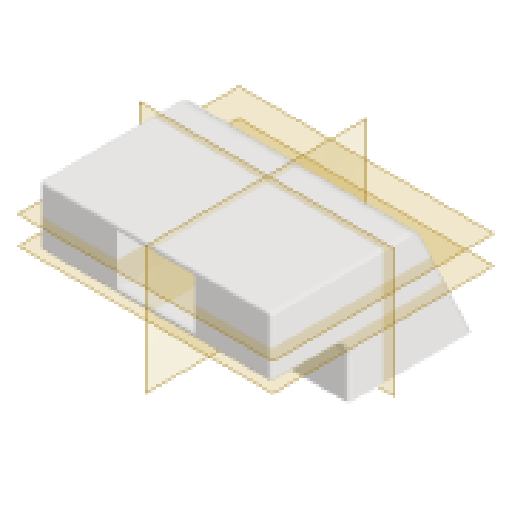
# Autodesk Inventor part: Вторая часть петли
Saved by Autodesk Inventor 2023.2 (Build 272271030, 271C)
## iProperties
Created: 2025-05-06
Part Number: Вторая часть петли
Material: Типовые
Document SubType Name: Modeling
Designer: Олег Коноваленко
Density: 1 g/cm^3
Appearance: По умолчанию
Author: Олег Коноваленко
Autodesk Inventor part; units mm, degrees
sketch "Эскиз1" plane through (0, 0, 0) normal (1, 0, 0) x (0, 1, 0)
  line L0 (-37.5, -57.5) -> (-37.5, 22.5)
  line L1 (-37.5, -57.5) -> (37.5, -22.5)
  line L2 (37.5, -22.5) -> (37.5, 22.5)
  line L3 (37.5, 22.5) -> (-37.5, 22.5)
  line L4 (37.5, -22.5) -> (-37.5, -22.5)
  line L5 (37.5, 22.5) -> (-37.5, -22.5) construction
  line L6 (37.5, -22.5) -> (-37.5, 22.5) construction
  line L7 (-52.5, 0) -> (52.5, 0) projected
  line L8 (0, 168.3234) -> (0, -95.1372) construction
  line L9 (18, 130.6862) -> (18, 46.6862) construction
  line L10 (37.5, 72.5) -> (37.5, 22.5)
  line L11 (-1.5, 72.5) -> (-1.5, 22.5)
  circle A0 centre (27.5, -16.1314) radius 10
  circle A1 centre (-11.5, 32.5) radius 10
  line L12 (37.5, 72.5) -> (-1.5, 72.5)
  point P0 (0, 0)
  point P1 (0, 0)
  point P2 (0, 0)
  point P3 (18, 88.6862)
  point P4 (0, 22.5)
  point P5 (19.7902, -22.5)
  point P6 (35.2098, -22.5)
  point P7 (37.5, -16.1314)
  point P8 (31.7289, -25.1932)
  point P9 (-1.5, 32.5)
  point P10 (-11.5, 22.5)
  dimension "d2" = 75
  dimension "d3" = 45
  dimension "d4" = 80
  dimension "d10" = 20
  dimension "d13" = 20
  dimension "d16" = 39
  dimension "d17" = 50
  constraints: 22 end point, 5 perpendicular, 4 midpoint, 4 tangent, 3 point on line, 3 vertical, 2 centre point, 2 other
  measures "d2" distance of L2.end L0.end
  measures "d3" distance of L1.end L2.end
  measures "d4" distance of L0.start L0.end
  measures "d10" diameter of A0
  measures "d13" diameter of A1
  measures "d16" distance of L11.start L10.start
  measures "d17" distance between parallel lines of L3 L12
extrude "Выдавливание2" add sketch "Эскиз1" along normal mid plane 150 contours L0 L4 A0 L1 | L0 L7 L2 A0 L4 | A0 L4 | L0 L3 L2 L7 | A0 L4 | A1 L11 L3 | L3 L11 L12 L10
fillet "Сопряжение1" radius 2 12 edges at (75, -1.5, 52.5) (75, -4.4289, 25.4289) (75, -24.5, 22.5) (75, 35.9347, -21.5031) (75, -2.8856, -41.3466) (75, 37.5, 28.1843) (-75, 35.9347, -21.5031) (-75, 37.5, 28.1843) (-75, -1.5, 52.5) (-75, -4.4289, 25.4289) (-75, -24.5, 22.5) (-75, -2.8856, -41.3466)
ref_plane "РабПлоскость1" through (-73, 18, 72.5) normal (0, 1, 0) x (1, 0, 0)
sketch "Эскиз7" plane through (-73, -1.5, 72.5) normal (0, 0, 1) x (1, 0, 0)
  line L0 (49, 34.5) -> (49, 4.5) construction
  line L1 (97, 4.5) -> (49, 4.5) construction
  line L2 (97, 34.5) -> (97, 4.5) construction
  line L3 (49, 34.5) -> (97, 34.5) construction
  line L4 (48.5, 4) -> (97.5, 4)
  line L5 (97.5, 4) -> (97.5, 35)
  line L6 (97.5, 35) -> (48.5, 35)
  line L7 (48.5, 35) -> (48.5, 4)
  line L8 (48.5, 4) -> (97.5, 35) construction
  line L9 (97.5, 4) -> (48.5, 35) construction
  point P0 (73, 1.5)
  point P1 (73, 19.5)
  dimension "d24" = 0.5
  dimension "d25" = 0.5
  dimension "d26" = 0.5
  dimension "d27" = 0.5
  constraints: 12 end point, 2 midpoint, 2 parallel, 1 horizontal, 1 perpendicular
  measures "d24" distance between parallel lines of L2 L5
  measures "d25" distance between parallel lines of L3 L6
  measures "d26" distance between parallel lines of L4 L1
  measures "d27" distance between parallel lines of L7 L0
extrude "Выдавливание6" cut sketch "Эскиз7" against normal blind 42.5
ref_plane "РабПлоскость2" through (24, 3, 30) normal (1, 0, 0) x (0, 1, 0)
ref_plane "РабПлоскость3" through (24, 3, 35.5) normal (1, 0, 0) x (0, 1, 0)
ref_plane "РабПлоскость4" through (-24, 3, 35.5) normal (-1, 0, 0) x (0, 0, 1)
fillet "Сопряжение2" radius 2 8 edges at (74.4142, 36.9142, 72.5) (75, 18, 72.5) (74.4142, -0.9142, 72.5) (0, -1.5, 72.5) (-74.4142, -0.9142, 72.5) (-75, 18, 72.5) (-74.4142, 36.9142, 72.5) (0, 37.5, 72.5)
chamfer "Фаска1" distance 1 angle 45 4 edges at (0, 33.5, 72.5) (-24.5, 18, 72.5) (0, 2.5, 72.5) (24.5, 18, 72.5)
sketch "Эскиз14" plane through (-73, -37.5, -57.5) normal (0, -1, 0) x (1, 0, 0)
  circle A0 centre (133, 70) radius 1.15
  line L0 (148, 78) -> (148, 2.2071) projected
  line L1 (0, 80) -> (146, 80) projected
  circle A1 centre (133, 55) radius 1.15
  circle A2 centre (133, 40) radius 1.15
  circle A3 centre (133, 25) radius 1.15
  circle A4 centre (133, 10) radius 1.15
  circle A5 centre (93, 70) radius 1.15
  circle A6 centre (93, 55) radius 1.15
  circle A7 centre (93, 40) radius 1.15
  circle A8 centre (93, 25) radius 1.15
  circle A9 centre (93, 10) radius 1.15
  circle A10 centre (53, 70) radius 1.15
  circle A11 centre (53, 55) radius 1.15
  circle A12 centre (53, 40) radius 1.15
  circle A13 centre (53, 25) radius 1.15
  circle A14 centre (53, 10) radius 1.15
  circle A15 centre (13, 70) radius 1.15
  circle A16 centre (13, 55) radius 1.15
  circle A17 centre (13, 40) radius 1.15
  circle A18 centre (13, 25) radius 1.15
  circle A19 centre (13, 10) radius 1.15
  point P0 (73, 57.5)
  dimension "d62" = 2.3
  dimension "d63" = 15
  dimension "d64" = 10
  dimension "d67" = 15
  dimension "d74" = 40
  constraints: 20 centre point, 1 horizontal, 1 vertical, 38 other
  measures "d62" diameter of A0
  measures "d63" distance from line of L0 A0.centre
  measures "d64" distance from line of L1 A0.centre
  measures "d67" distance of A0.centre A1.centre
  measures "d74" distance of A0.centre A5.centre
extrude "Выдавливание15" cut sketch "Эскиз14" against normal blind 10
